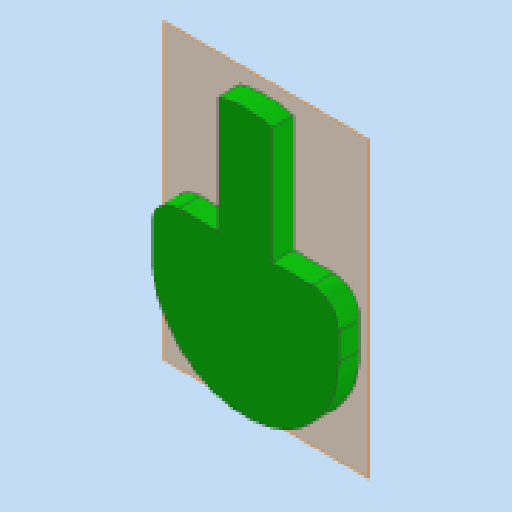
# Autodesk Inventor part: Sensor_PCB
Saved by Autodesk Inventor 2024 (Build 280153000, 153)
## iProperties
Created: 2025-02-15
Part Number: Sensor_PCB
Material: Generic
Document SubType Name: Modeling
Designer: XxPan
Density: 1 g/cm^3
Appearance: Default
Author: XxPan
Autodesk Inventor part; units mm, degrees
ref_plane "YZ Plane" through (0, 0, 0) normal (1, 0, 0) x (0, 1, 0)
ref_plane "XZ Plane" through (0, 0, 0) normal (0, 1, 0) x (-1, 0, 0)
ref_plane "XY Plane" through (0, 0, 0) normal (0, 0, 1) x (1, 0, 0)
sketch "Sketch1" plane through (0, 0, 0) normal (0, 0, 1) x (-1, 0, 0)
  line L0 (0, 0) -> (0, 6) construction
  line L1 (7, 0) -> (7, 6)
  line L2 (-7, 6) -> (-7, 0)
  arc A0 (-7, 0) -> (7, 0) centre (0, 0) ccw
  arc A1 (7, 6) -> (-7, 6) centre (0, 6) ccw
  point P0 (0, 3)
  dimension "d4" = 6
  dimension "d5" = 14
  constraints: 8 end point, 4 point on circle, 4 tangent, 2 centre point, 1 midpoint, 1 parallel, 1 vertical
  measures "d4" distance of L0.start L0.end
  measures "d5" diameter of A1
extrude "Extrusion1" add sketch "Sketch1" along normal blind 1.6
sketch "Sketch2" plane through (0, 0, 0) normal (0, 0, -1) x (-1, 0, 0)
  line L0 (-7, -6) -> (-7, 0) projected
  line L1 (-7, -2) -> (-2, -2)
  line L2 (-2, -2) -> (-2, 6.7082)
  arc A0 (7, 0) -> (-7, 0) centre (0, 0) ccw projected
  line L3 (7, -2) -> (2, -2)
  line L4 (2, -2) -> (2, 6.7082)
  line L5 (7, 0) -> (7, -6) projected
  line L6 (0, -17) -> (0, 11) construction
  line L7 (-9.8, 0) -> (9.8, 0) construction
  dimension "d6" = 4
  dimension "d7" = 2
  constraints: 8 end point, 3 point on line, 2 perpendicular, 2 point on circle, 1 horizontal, 1 other
  measures "d6" distance between parallel lines of L4 L2
  measures "d7" distance between parallel lines of L7 L1
extrude "Extrusion2" cut sketch "Sketch2" against normal up to surface (1.6 mm away)
fillet "Fillet1" radius 2 2 edges at (-7, -2, 0.8) (7, -2, 0.8)
body "Solid1"
